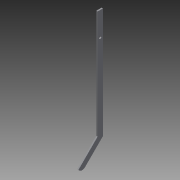
# Autodesk Inventor part: FlatArm
Saved by Autodesk Inventor 2013 (Build 170138000, 138)
## iProperties
Created: 2014-01-16
Part Number: FlatArm
Material: Generic
Document SubType Name: Modeling
Designer: 215152
Density: 1 g/cm^3
Author: 215152
Autodesk Inventor part; units mm, degrees
ref_plane "YZ Plane" through (0, 0, 0) normal (1, 0, 0) x (0, 1, 0)
ref_plane "XZ Plane" through (0, 0, 0) normal (0, 1, 0) x (-1, 0, 0)
ref_plane "XY Plane" through (0, 0, 0) normal (0, 0, 1) x (1, 0, 0)
sketch "Sketch1" plane through (0, 0, 0) normal (1, 0, 0) x (0, 1, 0)
  circle A0 centre (0, 0) radius 3.175
  line L0 (0, 0) -> (12.7, 0)
  line L1 (0, 0) -> (12.7, 0) construction
  line L2 (12.7, 0) -> (12.7, -12.7)
  line L3 (12.7, -12.7) -> (-405.9936, -12.7)
  line L4 (-405.9936, -12.7) -> (-405.9936, 12.7)
  line L5 (-405.9936, 12.7) -> (12.7, 12.7)
  line L6 (12.7, 12.7) -> (12.7, -12.7)
  line L7 (-405.9936, 12.7) -> (-498.3106, 105.017)
  line L8 (-405.9936, 12.7) -> (-275.4376, 12.7) construction
  line L9 (-498.3106, 105.017) -> (-516.2711, 87.0565)
  line L10 (-516.2711, 87.0565) -> (-408.5081, -20.7066)
  line L11 (-405.9936, -12.7) -> (-431.3936, -12.7)
  line L12 (-405.9936, -12.7) -> (-380.5936, -12.7) construction
  line L13 (-516.2711, 87.0565) -> (-416.5146, -12.7)
  line L14 (-416.5146, -12.7) -> (12.7, -12.7)
  dimension "d0" = 6.35
  dimension "d1" = 12.7
  dimension "d2" = 0
  dimension "d3" = 12.7
  dimension "d4" = 90
  dimension "d5" = 418.6936
  dimension "d6" = 25.4
  dimension "d7" = 130.556
  dimension "d8" = 135
  dimension "d9" = 25.4
  dimension "d10" = 90
  dimension "d11" = 152.4
  dimension "d12" = 90
  dimension "d13" = 25.4
  dimension "d14" = 180
  constraints: 30 end point, 5 horizontal, 4 parallel, 4 perpendicular, 3 equal length, 2 point on line, 1 centre point, 1 coincident
  measures "d0" diameter of A0
  measures "d1" distance of L0.start L0.end
  measures "d2" distance between parallel lines of L0 L1
  measures "d3" distance of L0.end L2.end
  measures "d4" angle of L0 L2
  measures "d5" distance of L4.end L5.end
  measures "d6" distance of L3.end L4.end
  measures "d7" distance of L4.end L7.end
  measures "d8" angle of L8 L7
  measures "d9" distance of L7.end L9.end
  measures "d10" angle of L9 L7
  measures "d11" distance of L9.end L10.end
  measures "d12" angle of L10 L9
  measures "d13" distance of L3.end L11.end
  measures "d14" angle of L11 L12
extrude "Extrusion1" add sketch "Sketch1" along normal blind 25.4
sketch "Sketch2" plane through (25.4, 0, 0) normal (1, 0, 0) x (0, 0, -1)
  line L0 (-105.017, -498.3106) -> (-87.0565, -516.2711) projected
  line L1 (-87.0565, -516.2711) -> (12.7, -416.5146) projected
  line L2 (-12.7, 12.7) -> (-12.7, -405.9936) projected
  line L3 (-96.0368, -507.2909) -> (-78.0763, -507.2909)
  line L4 (-105.017, -498.3106) -> (-100.5269, -502.8008)
  line L5 (-100.5269, -502.8008) -> (-73.5861, -502.8008)
  arc A0 (-100.5269, -502.8008) -> (-73.5861, -502.8008) centre (-87.0565, -489.3304) ccw
  dimension "d17" = 6.35
  dimension "d18" = 19.05
  constraints: 6 end point, 3 point on line, 2 point on circle, 1 centre point, 1 midpoint, 1 parallel, 1 perpendicular
  measures "d17" distance of L0.start L4.end
  measures "d18" radius of A0
extrude "Extrusion2" cut sketch "Sketch2" against normal blind 25.4 contours A0 L3 L0 | L3 A0 L1 L0 | L1 L3 A0
sketch "Sketch3" plane through (0, 12.7, 12.7) normal (0, 1, 0) x (1, 0, 0)
  line L0 (0, 25.4) -> (0, 0) projected
  line L1 (0, 0) -> (25.4, 0) projected
  line L2 (25.4, 25.4) -> (25.4, 0) projected
  line L3 (0, 25.4) -> (25.4, 25.4) projected
  point P0 (0, 12.7)
extrude "Extrusion3" add sketch "Sketch3" along normal blind 127
sketch "Sketch4" plane through (25.4, 0, 0) normal (1, 0, 0) x (0, 0, -1)
  arc A0 (-100.5269, -502.8008) -> (-73.5861, -502.8008) centre (-87.0565, -489.3304) ccw projected
  line L0 (-73.5861, -502.8008) -> (12.7, -416.5146) projected
  line L1 (12.7, -416.5146) -> (12.7, 139.7) projected
  line L2 (-12.7, 139.7) -> (12.7, 139.7) projected
  line L3 (-12.7, -405.9936) -> (-12.7, 139.7) projected
  line L4 (-12.7, -405.9936) -> (-105.017, -498.3106) projected
  line L5 (-105.017, -498.3106) -> (-100.5269, -502.8008) projected
  circle A1 centre (0, 0) radius 3.175 projected
extrude "Extrusion4" cut sketch "Sketch4" against normal blind 19.05
sketch "Sketch5" plane through (6.35, 0, 0) normal (1, 0, 0) x (0, 0, -1)
  line L0 (-12.7, 139.7) -> (12.7, 139.7)
  line L1 (12.7, 139.7) -> (12.7, 12.7)
  line L2 (12.7, 12.7) -> (-12.7, 12.7)
  line L3 (-12.7, 12.7) -> (-12.7, 139.7)
  dimension "d25" = 25.4
  dimension "d26" = 127
  constraints: 8 end point, 2 parallel, 1 horizontal, 1 perpendicular
  measures "d25" distance of L1.end L2.end
  measures "d26" distance of L0.end L1.end
extrude "Extrusion5" cut sketch "Sketch5" against normal blind 127
sketch "Sketch8" plane through (6.35, 12.7, 12.7) normal (0, 1, 0) x (1, 0, 0)
  line L0 (-6.35, 0) -> (-6.35, 25.4) projected
  line L1 (0, 0) -> (-6.35, 0) projected
  line L2 (0, 25.4) -> (0, 0) projected
  line L3 (-6.35, 25.4) -> (0, 25.4) projected
  point P0 (-6.35, 12.7)
extrude "Extrusion8" add sketch "Sketch8" along normal blind 101.6
sketch "Sketch9" plane through (6.35, 0, 0) normal (1, 0, 0) x (0, 0, -1)
  circle A0 centre (0, 0) radius 3.175 projected
  circle A1 centre (0, 0) radius 6.35
  dimension "d45" = 12.7
  constraints: 1 centre point, 1 coincident
  measures "d45" diameter of A1
extrude "Extrusion9" cut sketch "Sketch9" against normal blind 25.4
sketch "Sketch10" plane through (6.35, 0, 0) normal (1, 0, 0) x (0, 0, -1)
  circle A0 centre (0, 0) radius 6.35 projected
  line L0 (-5.5563, -5.5563) -> (5.5563, -5.5563)
  line L1 (5.5563, -5.5563) -> (5.5563, 5.5563)
  line L2 (5.5563, 5.5563) -> (-5.5563, 5.5563)
  line L3 (-5.5563, 5.5563) -> (-5.5563, -5.5563)
  line L4 (-5.5563, -5.5563) -> (5.5563, 5.5563) construction
  line L5 (5.5563, -5.5563) -> (-5.5563, 5.5563) construction
  line L6 (5.5563, -3.0742) -> (0.1158, -6.3489)
  line L7 (0.1158, -6.3489) -> (-5.4404, -3.2748)
  line L8 (-5.4404, -3.2748) -> (-5.5563, 3.0742)
  line L9 (-5.5563, 3.0742) -> (-0.1158, 6.3489)
  line L10 (-0.1158, 6.3489) -> (5.4404, 3.2748)
  line L11 (5.4404, 3.2748) -> (5.5563, -3.0742)
  dimension "d48" = 11.1125
  dimension "d49" = 11.1125
  constraints: 24 end point, 2 midpoint, 2 parallel, 1 coincident, 1 horizontal, 1 perpendicular, 1 point on line, 15 other
  measures "d48" distance of L2.end L1.end
  measures "d49" distance of L1.end L0.end
extrude "Extrusion10" add sketch "Sketch10" against normal blind 6.35 contours L1 A0 | L11 A0 L1 | A0 L0 L6 | A0 L6 L0 | L10 L2 A0 | A0 L0 L7 | L0 A0 L7 | L2 L10 A0 | A0 L3 L8 | L9 L2 A0 | L9 A0 L2 | A0 L3
body "Solid1"
